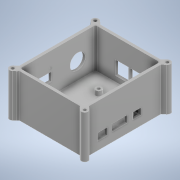
# Autodesk Inventor part: Case Rev D
Saved by Autodesk Inventor 2021 (Build 250183000, 183)
## iProperties
Created: 2021-07-24
Part Number: Case Rev D
Material: ABS Plastic
Document SubType Name: Modeling
Designer: cmzgt
Density: 0.1 g/cm^3
Appearance: Smooth - White
Author: cmzgt
## iProperties of the stored document _3DPrint.ipt
Created: 2021-08-03
Part Number: _3DPrint
Material: Generic
Document SubType Name: Modeling
Designer: cmzgt
Density: 1 g/cm^3
Appearance: Default
Author: cmzgt
Autodesk Inventor part; units mm, degrees
ref_plane "YZ Plane" through (0, 0, 0) normal (1, 0, 0) x (0, 1, 0)
ref_plane "XZ Plane" through (0, 0, 0) normal (0, 1, 0) x (-1, 0, 0)
ref_plane "XY Plane" through (0, 0, 0) normal (0, 0, 1) x (1, 0, 0)
sketch "Sketch1" plane through (0, 0, 0) normal (0, 1, 0) x (-1, 0, 0)
  line L0 (-43.3, -50.05) -> (43.3, -50.05)
  line L1 (43.3, -50.05) -> (43.3, 50.05)
  line L2 (43.3, 50.05) -> (-43.3, 50.05)
  line L3 (-43.3, 50.05) -> (-43.3, -50.05)
  line L4 (-43.3, -50.05) -> (43.3, 50.05) construction
  line L5 (43.3, -50.05) -> (-43.3, 50.05) construction
  point P0 (0, 0)
  dimension "d0" = 86.6
  dimension "d1" = 100.1
  constraints: 12 end point, 2 midpoint, 2 parallel, 1 horizontal, 1 perpendicular
  measures "d0" distance of L2.end L1.end
  measures "d1" distance of L0.end L1.end
extrude "Extrusion1" add sketch "Sketch1" along normal blind 4.445
sketch "Sketch2" plane through (0, 4.445, 0) normal (0, 1, 0) x (1, 0, 0)
  line L0 (40.1, 46.85) -> (-40.1, 46.85)
  line L1 (-40.1, 46.85) -> (-40.1, -46.85)
  line L2 (-40.1, -46.85) -> (40.1, -46.85)
  line L3 (40.1, -46.85) -> (40.1, 46.85)
  line L4 (40.1, 46.85) -> (-40.1, -46.85) construction
  line L5 (-40.1, 46.85) -> (40.1, -46.85) construction
  line L6 (-43.3, 50.05) -> (-43.3, -50.05) projected
  line L7 (-43.3, -50.05) -> (43.3, -50.05) projected
  line L8 (43.3, 50.05) -> (-43.3, 50.05) projected
  line L9 (43.3, -50.05) -> (43.3, 50.05) projected
  line L10 (36.9, -43.65) -> (43.3, -50.05) construction
  line L11 (34.4431, -46.85) -> (40.4716, -52.8784)
  line L12 (46.1284, -47.2216) -> (40.1, -41.1931)
  arc A0 (40.4716, -52.8784) -> (46.1284, -47.2216) centre (43.3, -50.05) ccw
  circle A1 centre (43.3, -50.05) radius 1.375
  point P0 (0, 0)
  dimension "d4" = 3.2
  dimension "d5" = 3.2
  dimension "d22" = 8
  dimension "d23" = 2.75
  constraints: 20 end point, 4 parallel, 3 midpoint, 2 centre point, 2 point on circle, 2 point on line, 2 tangent, 1 coincident, 1 horizontal, 1 perpendicular
  measures "d4" distance between parallel lines of L6 L1
  measures "d5" distance between parallel lines of L7 L2
  measures "d22" diameter of A0
  measures "d23" diameter of A1
extrude "Extrusion2" add sketch "Sketch2" along normal blind 49 contours L0 L1 L2 L11 L7 L6 L8 L9 L12 L3 | L12 L9 A1 L7 L11 L2 L3 | L9 L7 A1 picked at (42.4402, -49.7491)
sketch "Sketch4" plane through (0, 0, 0) normal (0, -1, 0) x (1, 0, 0)
  line L0 (41.7906, 48.7379) -> (44.8094, 51.3621) construction
  line L1 (43.3, 50.05) -> (43.3, -50.05) projected
  line L2 (43.3, 44.7499) -> (47.4337, 48.3433)
  line L3 (42.1852, 54.381) -> (39.1663, 51.7567)
  arc A0 (39.1663, 51.7567) -> (38.0119, 50.05) centre (41.7906, 48.7379) ccw
  arc A1 (47.4337, 48.3433) -> (42.1852, 54.381) centre (44.8094, 51.3621) ccw
  line L4 (-43.3, 50.05) -> (43.3, 50.05) projected
  line L5 (38.0119, 50.05) -> (43.3, 50.05)
  line L6 (43.3, 50.05) -> (43.3, 44.7499)
  circle A2 centre (44.8094, 51.3621) radius 1.985
  line L7 (0, 50.05) -> (0, -50.05) construction
  line L8 (43.3, -50.05) -> (-43.3, -50.05) construction
  line L9 (43.3, 0) -> (-33.3, 0) construction
  line L10 (43.3, -50.05) -> (43.3, 50.05)
  line L11 (43.3, -44.7499) -> (47.4337, -48.3433)
  line L12 (42.1852, -54.381) -> (39.1663, -51.7567)
  arc A3 (38.0119, -50.05) -> (39.1663, -51.7567) centre (41.7906, -48.7379) ccw
  arc A4 (42.1852, -54.381) -> (47.4337, -48.3433) centre (44.8094, -51.3621) ccw
  line L13 (-43.3, -50.05) -> (43.3, -50.05)
  circle A5 centre (44.8094, -51.3621) radius 1.985
  line L14 (-43.3, 50.05) -> (-43.3, -50.05)
  line L15 (-43.3, 44.7499) -> (-47.4337, 48.3433)
  line L16 (-42.1852, 54.381) -> (-39.1663, 51.7567)
  arc A6 (-38.0119, 50.05) -> (-39.1663, 51.7567) centre (-41.7906, 48.7379) ccw
  arc A7 (-42.1852, 54.381) -> (-47.4337, 48.3433) centre (-44.8094, 51.3621) ccw
  line L17 (-38.0119, 50.05) -> (-43.3, 50.05)
  circle A8 centre (-44.8094, 51.3621) radius 1.985
  arc A9 (-47.4337, -48.3433) -> (-42.1852, -54.381) centre (-44.8094, -51.3621) ccw
  line L18 (-43.3, -44.7499) -> (-47.4337, -48.3433)
  line L19 (-42.1852, -54.381) -> (-39.1663, -51.7567)
  arc A10 (-39.1663, -51.7567) -> (-38.0119, -50.05) centre (-41.7906, -48.7379) ccw
  circle A11 centre (-44.8094, -51.3621) radius 1.985
  line L20 (-38.0119, -50.05) -> (-43.3, -50.05)
  line L21 (-43.3, -50.05) -> (-43.3, 50.05)
  point P0 (0, 0)
  point P1 (-38.0119, -50.05)
  point P2 (-43.3, -44.7499)
  point P3 (-38.0119, 50.05)
  point P4 (43.3, -44.7499)
  point P5 (43.3, -50.05)
  dimension "d24" = 2
  dimension "d25" = 8
  dimension "d26" = 131
  dimension "d27" = 3.97
  constraints: 40 end point, 30 symmetric about line, 16 point on circle, 12 centre point, 6 point on line, 4 coincident, 4 midpoint, 4 tangent, 1 collinear, 1 horizontal, 1 parallel, 9 other
  measures "d24" distance of L1.start L0.end
  measures "d25" diameter of A1
  measures "d26" angle of L1 L2
  measures "d27" diameter of A2
extrude "Extrusion4" add sketch "Sketch4" against normal up to surface (53.445 mm away) contours L4 A0 L3 A1 L2 L1 | L11 A4 L12 A3 L13 L1 | L4 L14 L15 A7 L16 A6 | A10 L19 A9 L18 L14 L13
fillet "Fillet2" radius 2 4 edges at (40.1, 28.945, -46.85) (-40.1, 28.945, -46.85) (-40.1, 28.945, 46.85) (40.1, 28.945, 46.85)
sketch "Sketch14" plane through (0, 4.445, 0) normal (0, 1, 0) x (1, 0, 0)
  circle A0 centre (36.6, -34.85) radius 3.7
  circle A1 centre (36.6, -34.85) radius 1.985
  line L0 (38.1, -46.85) -> (-38.1, -46.85) projected
  line L1 (40.1, 44.85) -> (40.1, -44.85) projected
  line L2 (-38.1, -46.85) -> (38.1, -46.85) construction
  line L3 (0, -46.85) -> (0, 50.05) construction
  line L4 (38.0119, 50.05) -> (-38.0119, 50.05) construction
  circle A2 centre (36.6, 23.15) radius 3.7
  circle A3 centre (36.6, 23.15) radius 1.985
  line L5 (-40.1, 44.85) -> (-40.1, -44.85) construction
  line L6 (-40.1, 0) -> (40.1, 0) construction
  line L7 (40.1, -44.85) -> (40.1, 44.85) construction
  circle A4 centre (-12.4, -34.85) radius 3.7
  circle A5 centre (-12.4, -34.85) radius 1.985
  circle A6 centre (-12.4, 23.15) radius 1.985
  circle A7 centre (-12.4, 23.15) radius 3.7
  point P0 (0, 0)
  dimension "d114" = 7.4
  dimension "d115" = 3.97
  dimension "d116" = 12
  dimension "d117" = 3.5
  dimension "d120" = 58
  dimension "d127" = 49
  constraints: 8 centre point, 4 coincident, 4 end point, 4 midpoint, 1 horizontal, 1 vertical, 12 other
  measures "d114" diameter of A0
  measures "d115" diameter of A1
  measures "d116" distance from line of L0 A0.centre
  measures "d117" distance from line of L1 A0.centre
  measures "d120" distance of A0.centre A2.centre
  measures "d127" distance of A0.centre A4.centre
sketch "Sketch15" plane through (0, 4.445, 0) normal (0, 1, 0) x (1, 0, 0)
  point P0 (0, 0)
extrude "Extrusion10" add sketch "Sketch14" along normal blind 6
sketch "Sketch16" plane through (43.3, 0, 44.7499) normal (1, 0, 0) x (0, 0, -1)
  line L0 (12.9515, 13.2621) -> (12.9515, 13.455) projected
  line L1 (20.9323, 13.455) -> (20.9323, 13.2621) projected
  line L2 (13.9419, 14.5004) -> (19.9419, 14.5004) projected
  line L3 (88.3241, 11.975) -> (9.3999, 11.975) projected
  line L4 (22.9323, 9.975) -> (10.9515, 9.975)
  line L5 (10.9515, 9.975) -> (10.9515, 19.0004)
  line L6 (10.9515, 19.0004) -> (22.9323, 19.0004)
  line L7 (22.9323, 19.0004) -> (22.9323, 9.975)
  line L8 (30.8419, 17.055) -> (30.8419, 14.5766) projected
  line L9 (45.8419, 14.5766) -> (45.8419, 17.055) projected
  line L10 (45.0419, 17.855) -> (31.6419, 17.855) projected
  line L11 (47.8419, 10.975) -> (28.8419, 10.975)
  line L12 (28.8419, 10.975) -> (28.8419, 19.855)
  line L13 (28.8419, 19.855) -> (47.8419, 19.855)
  line L14 (47.8419, 19.855) -> (47.8419, 10.975)
  line L15 (56.4419, 17.775) -> (56.4419, 11.775) projected
  line L16 (63.4419, 11.775) -> (63.4419, 17.775) projected
  line L17 (63.4419, 17.775) -> (59.9419, 17.775) projected
  line L18 (59.9419, 17.775) -> (56.4419, 17.775) projected
  line L19 (64.9419, 10.975) -> (54.9419, 10.975)
  line L20 (54.9419, 10.975) -> (54.9419, 19.275)
  line L21 (54.9419, 19.275) -> (64.9419, 19.275)
  line L22 (64.9419, 19.275) -> (64.9419, 10.975)
  point P0 (44.7499, 0)
  dimension "d134" = 4.5
  dimension "d135" = 2
  dimension "d136" = 2
  dimension "d137" = 2
  dimension "d138" = 2
  dimension "d139" = 1
  dimension "d140" = 2
  dimension "d141" = 2
  dimension "d142" = 1
  dimension "d143" = 1.5
  dimension "d144" = 1.5
  dimension "d145" = 1.5
  constraints: 24 end point, 6 parallel, 3 horizontal, 3 perpendicular
  measures "d134" distance between parallel lines of L2 L6
  measures "d135" distance between parallel lines of L3 L4
  measures "d136" distance between parallel lines of L1 L7
  measures "d137" distance between parallel lines of L5 L0
  measures "d138" distance between parallel lines of L13 L10
  measures "d139" distance between parallel lines of L3 L11
  measures "d140" distance between parallel lines of L9 L14
  measures "d141" distance from line of L8.end L12
  measures "d142" distance between parallel lines of L3 L19
  measures "d143" distance between parallel lines of L16 L22
  measures "d144" distance between parallel lines of L15 L20
  measures "d145" distance between parallel lines of L18 L21
extrude "Extrusion11" cut sketch "Sketch16" against normal up to surface (3.2 mm away)
sketch "Sketch17" plane through (38.0119, 0, -50.05) normal (0, 0, -1) x (-1, 0, 0)
  line L0 (16.1912, 11.975) -> (16.1912, 25.475) projected
  line L1 (0.3112, 11.975) -> (0.3112, 25.475) projected
  line L2 (0.3112, 25.475) -> (16.1912, 25.475) projected
  line L3 (50.9119, 11.975) -> (0.9119, 11.975) projected
  line L4 (16.4912, 11.725) -> (0.0112, 11.725)
  line L5 (0.0112, 11.725) -> (0.0112, 25.725)
  line L6 (0.0112, 25.725) -> (16.4912, 25.725)
  line L7 (16.4912, 25.725) -> (16.4912, 11.725)
  line L8 (19.4512, 18.7546) -> (19.4512, 21.7546) projected
  line L9 (34.5512, 21.7546) -> (34.5512, 18.7546) projected
  line L10 (24.0012, 27.465) -> (30.0012, 27.465) projected
  line L11 (35.2512, 11.225) -> (18.7512, 11.225)
  line L12 (18.7512, 11.225) -> (18.7512, 28.465)
  line L13 (18.7512, 28.465) -> (35.2512, 28.465)
  line L14 (35.2512, 28.465) -> (35.2512, 11.225)
  line L15 (37.4512, 18.7546) -> (37.4512, 21.7546) projected
  line L16 (52.5512, 21.7546) -> (52.5512, 18.7546) projected
  line L17 (42.0012, 27.465) -> (48.0012, 27.465) projected
  line L18 (53.2512, 11.225) -> (36.7512, 11.225)
  line L19 (36.7512, 11.225) -> (36.7512, 28.465)
  line L20 (36.7512, 28.465) -> (53.2512, 28.465)
  line L21 (53.2512, 28.465) -> (53.2512, 11.225)
  point P0 (38.0119, 0)
  point P1 (18.7512, 11.975)
  point P2 (35.2512, 11.975)
  dimension "d148" = 0.3
  dimension "d149" = 0.3
  dimension "d150" = 0.25
  dimension "d151" = 0.25
  dimension "d154" = 0.7
  dimension "d155" = 0.7
  dimension "d156" = 1
  dimension "d157" = 0.75
  dimension "d158" = 1
  dimension "d159" = 0.7
  dimension "d160" = 0.7
  dimension "d161" = 0.75
  constraints: 24 end point, 6 parallel, 3 horizontal, 3 perpendicular
  measures "d148" distance between parallel lines of L1 L5
  measures "d149" distance between parallel lines of L0 L7
  measures "d150" distance between parallel lines of L3 L4
  measures "d151" distance between parallel lines of L2 L6
  measures "d154" distance between parallel lines of L8 L12
  measures "d155" distance between parallel lines of L9 L14
  measures "d156" distance between parallel lines of L10 L13
  measures "d157" distance between parallel lines of L3 L11
  measures "d158" distance between parallel lines of L17 L20
  measures "d159" distance between parallel lines of L15 L19
  measures "d160" distance between parallel lines of L21 L16
  measures "d161" distance between parallel lines of L3 L18
extrude "Extrusion12" cut sketch "Sketch17" against normal up to surface (3.2 mm away)
sketch "Sketch19" plane through (-43.3, 0, -44.7499) normal (-1, 0, 0) x (0, 0, 1)
  circle A0 centre (20, 25) radius 9.6
  line L0 (0, 53.445) -> (0, 0) projected
  line L1 (0, 0) -> (89.4999, 0) projected
  point P0 (44.7499, 0)
  dimension "d162" = 19.2
  dimension "d163" = 20
  dimension "d164" = 25
  constraints: 1 centre point
  measures "d162" diameter of A0
  measures "d163" distance from line of L0 A0.centre
  measures "d164" distance from line of L1 A0.centre
extrude "Extrusion13" cut sketch "Sketch19" against normal up to surface (3.2 mm away)
sketch "Sketch23" plane through (-43.3, 0, -44.7499) normal (-1, 0, 0) x (0, 0, 1)
  line L0 (52.1999, 9.1) -> (79.4999, 9.1)
  line L1 (79.4999, 9.1) -> (79.4999, 36.9)
  line L2 (79.4999, 36.9) -> (52.1999, 36.9)
  line L3 (52.1999, 36.9) -> (52.1999, 9.1)
  line L4 (89.4999, 0) -> (89.4999, 53.445) projected
  line L5 (0, 0) -> (89.4999, 0) projected
  circle A0 centre (54.1999, 34.9) radius 1
  line L6 (65.8499, 36.9) -> (65.8499, 9.1) construction
  line L7 (52.1999, 23) -> (79.4999, 23) construction
  circle A1 centre (77.4999, 34.9) radius 1
  circle A2 centre (54.1999, 11.1) radius 1
  circle A3 centre (77.4999, 11.1) radius 1
  line L8 (78.8499, 19.53) -> (52.8499, 19.53)
  line L9 (52.8499, 19.53) -> (52.8499, 30.53)
  line L10 (52.8499, 30.53) -> (78.8499, 30.53)
  line L11 (78.8499, 30.53) -> (78.8499, 19.53)
  line L12 (78.8499, 19.53) -> (52.8499, 30.53) construction
  line L13 (52.8499, 19.53) -> (78.8499, 30.53) construction
  line L14 (79.1999, 13.37) -> (52.4999, 13.37)
  line L15 (52.4999, 13.37) -> (52.4999, 32.63)
  line L16 (52.4999, 32.63) -> (79.1999, 32.63)
  line L17 (79.1999, 32.63) -> (79.1999, 13.37)
  line L18 (79.1999, 13.37) -> (52.4999, 32.63) construction
  line L19 (52.4999, 13.37) -> (79.1999, 32.63) construction
  point P0 (44.7499, 0)
  point P1 (65.8499, 25.03)
  point P2 (65.8499, 23)
  dimension "d208" = 27.3
  dimension "d209" = 27.8
  dimension "d210" = 10
  dimension "d212" = 2
  dimension "d213" = 2
  dimension "d214" = 2
  dimension "d215" = 26
  dimension "d216" = 11
  dimension "d217" = 6.37
  dimension "d218" = 26.7
  dimension "d219" = 19.26
  dimension "d220" = 4.27
  dimension "d223" = 23
  constraints: 36 end point, 9 midpoint, 6 parallel, 4 centre point, 3 horizontal, 3 perpendicular, 3 symmetric about line, 1 point on line, 3 other
  measures "d208" distance of L2.end L1.end
  measures "d209" distance of L1.end L0.end
  measures "d210" distance between parallel lines of L4 L1
  measures "d212" diameter of A0
  measures "d213" distance from line of L2 A0.centre
  measures "d214" distance from line of L3 A0.centre
  measures "d215" distance of L9.end L10.end
  measures "d216" distance of L8.end L9.end
  measures "d217" distance between parallel lines of L2 L10
  measures "d218" distance of L15.end L16.end
  measures "d219" distance of L14.end L15.end
  measures "d220" distance between parallel lines of L2 L16
  measures "d223" distance between parallel lines of L5 L7
extrude "Extrusion17" cut sketch "Sketch23" against normal up to surface (3.2 mm away) contours A0 | A1 | A2 | A3 | L8 L9 L10 L11
body "Solid1"
